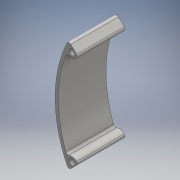
# Autodesk Inventor part: back plate
Saved by Autodesk Inventor 2016 (Build 200138000, 138)
## iProperties
Created: 2015-10-26
Part Number: back plate
Material: Generic
Document SubType Name: Modeling
Designer: Hulbert Office
Density: 1 g/cm^3
Appearance: Default
Author: Hulbert Office
Autodesk Inventor part; units mm, degrees
ref_plane "YZ Plane" through (0, 0, 0) normal (1, 0, 0) x (0, 1, 0)
ref_plane "XZ Plane" through (0, 0, 0) normal (0, 1, 0) x (-1, 0, 0)
ref_plane "XY Plane" through (0, 0, 0) normal (0, 0, 1) x (1, 0, 0)
sketch "Sketch1" plane through (0, 0, 0) normal (0, 1, 0) x (-1, 0, 0)
  line L0 (-57.8698, 32.3928) -> (-57.8698, 32.0292)
  line L1 (-57.8698, 32.0292) -> (-57.8698, 18.4092)
  line L2 (-57.8698, 18.4092) -> (-57.8698, 4.7892)
  line L3 (-57.8698, 4.7892) -> (-57.8698, -8.8308)
  line L4 (-57.8698, -8.8308) -> (-57.8698, -22.4508)
  line L5 (-57.8698, -1.839) -> (-57.8698, -36.0708)
  line L6 (-57.8698, -36.0708) -> (-54.7847, -36.7468)
  line L7 (-54.7847, -36.7468) -> (-50.239, -34.4141)
  line L8 (-50.239, -34.4141) -> (-38.1725, -14.554)
  line L9 (-38.1725, -14.554) -> (-34.8422, -12.8451)
  line L10 (-34.8422, -12.8451) -> (-8.0341, -30.0588)
  line L11 (-8.0341, -30.0588) -> (-8.0341, -78.5822)
  line L12 (-8.0341, -78.5822) -> (-8.0341, -99.6831)
  line L13 (-8.0341, -99.6831) -> (-7.0952, -101.449)
  line L14 (-7.0952, -101.449) -> (-2.0952, -101.449)
  line L15 (-1.1562, -99.6831) -> (-2.0952, -101.449)
  line L16 (-1.1562, -78.5822) -> (-1.1562, -99.6831)
  line L17 (-1.1562, -30.0588) -> (-1.1562, -78.5822)
  line L18 (-1.1562, -30.0588) -> (21.4276, -7.475)
  line L19 (21.4276, -7.475) -> (24.147, -4.7556)
  line L20 (24.147, -4.7556) -> (89.8399, -4.7556)
  line L21 (89.8399, -4.7556) -> (91.6058, -3.8166)
  line L22 (91.6058, 0.1386) -> (91.6058, -3.8166)
  line L23 (89.8399, 1.0776) -> (91.6058, 0.1386)
  line L24 (24.147, 1.0776) -> (89.8399, 1.0776)
  line L25 (21.4276, 3.797) -> (24.147, 1.0776)
  line L26 (-1.1562, 26.3808) -> (21.4276, 3.797)
  line L27 (-1.1562, 26.3808) -> (-1.1562, 74.9042)
  line L28 (-1.1562, 74.9042) -> (-1.1562, 96.0051)
  line L29 (-1.1562, 96.0051) -> (-2.0952, 97.771)
  line L30 (-7.0952, 97.771) -> (-2.0952, 97.771)
  line L31 (-8.0341, 96.0051) -> (-7.0952, 97.771)
  line L32 (-8.0341, 74.9042) -> (-8.0341, 96.0051)
  line L33 (-8.0341, 74.9042) -> (-8.0341, 96.0051)
  line L34 (-8.0341, 26.3808) -> (-8.0341, 74.9042)
  line L35 (-8.0341, 26.3808) -> (-8.0341, 74.9042)
  line L36 (-8.0341, 26.3808) -> (-8.0341, 74.9042)
  line L37 (-8.0341, 26.3808) -> (-8.0341, 74.9042)
  line L38 (-34.8422, 9.1671) -> (-8.0341, 26.3808)
  line L39 (-38.1725, 10.876) -> (-34.8422, 9.1671)
  line L40 (-50.239, 30.7361) -> (-38.1725, 10.876)
  line L41 (-54.7847, 33.0688) -> (-50.239, 30.7361)
  line L42 (-57.8698, 32.3928) -> (-54.7847, 33.0688)
  line L43 (-57.8698, -1.839) -> (-57.8698, -36.0708)
  line L44 (-57.8698, -1.839) -> (-57.8698, -36.0708)
  line L45 (-57.8698, -1.839) -> (-57.8698, -36.0708)
  line L46 (-57.8698, -36.0708) -> (-54.7847, -36.7468)
  line L47 (-54.7847, -36.7468) -> (-50.239, -34.4141)
  line L48 (-50.239, -34.4141) -> (-38.1725, -14.554)
  line L49 (-38.1725, -14.554) -> (-34.8422, -12.8451)
  line L50 (-34.8422, -12.8451) -> (-8.0341, -30.0588)
  line L51 (-8.0341, -30.0588) -> (-8.0341, -78.5822)
  line L52 (-8.0341, -78.5822) -> (-8.0341, -99.6831)
  line L53 (-8.0341, -99.6831) -> (-7.0952, -101.449)
  line L54 (-7.0952, -101.449) -> (-2.0952, -101.449)
  line L55 (-1.1562, -99.6831) -> (-2.0952, -101.449)
  line L56 (-1.1562, -78.5822) -> (-1.1562, -99.6831)
  line L57 (-1.1562, -30.0588) -> (-1.1562, -78.5822)
  line L58 (-1.1562, -30.0588) -> (21.4276, -7.475)
  line L59 (21.4276, -7.475) -> (24.147, -4.7556)
  line L60 (24.147, -4.7556) -> (89.8399, -4.7556)
  line L61 (89.8399, -4.7556) -> (91.6058, -3.8166)
  line L62 (91.6058, 0.1386) -> (91.6058, -3.8166)
  line L63 (89.8399, 1.0776) -> (91.6058, 0.1386)
  line L64 (24.147, 1.0776) -> (89.8399, 1.0776)
  line L65 (21.4276, 3.797) -> (24.147, 1.0776)
  line L66 (-1.1562, 26.3808) -> (21.4276, 3.797)
  line L67 (-1.1562, 26.3808) -> (-1.1562, 74.9042)
  line L68 (-1.1562, 74.9042) -> (-1.1562, 96.0051)
  line L69 (-1.1562, 96.0051) -> (-2.0952, 97.771)
  line L70 (-7.0952, 97.771) -> (-2.0952, 97.771)
  line L71 (-8.0341, 96.0051) -> (-7.0952, 97.771)
  line L72 (-8.0341, 74.9042) -> (-8.0341, 96.0051)
  line L73 (-8.0341, 69.2148) -> (-8.0341, 83.4928)
  line L74 (-8.0341, 54.9368) -> (-8.0341, 69.2148)
  line L75 (-8.0341, 40.6588) -> (-8.0341, 54.9368)
  line L76 (-8.0341, 26.3808) -> (-8.0341, 40.6588)
  line L77 (-34.8422, 9.1671) -> (-8.0341, 26.3808)
  line L78 (-38.1725, 10.876) -> (-34.8422, 9.1671)
  line L79 (-50.239, 30.7361) -> (-38.1725, 10.876)
  line L80 (-54.7847, 33.0688) -> (-50.239, 30.7361)
  line L81 (-57.8698, 32.3928) -> (-54.7847, 33.0688)
  line L82 (-57.8698, 32.3928) -> (-57.8698, 32.0292)
  line L83 (-57.8698, 32.0292) -> (-57.8698, 18.4092)
  line L84 (-57.8698, -1.839) -> (-57.8698, 26.3808)
  line L85 (-57.8698, -1.839) -> (-57.8698, 26.3808)
  line L86 (-8.0341, 26.3808) -> (-8.0341, 40.6588)
  line L87 (-34.8422, 9.1671) -> (-8.0341, 26.3808)
  line L88 (-38.1725, 10.876) -> (-34.8422, 9.1671)
  line L89 (-50.239, 30.7361) -> (-38.1725, 10.876)
  line L90 (-54.7847, 33.0688) -> (-50.239, 30.7361)
  line L91 (-57.8698, 32.3928) -> (-54.7847, 33.0688)
  line L92 (-57.8698, 32.3928) -> (-57.8698, 32.0292)
  line L93 (-57.8698, 32.0292) -> (-57.8698, 18.4092)
  line L94 (-57.8698, -1.839) -> (-57.8698, 26.3808)
  line L95 (-57.8698, -1.839) -> (-57.8698, 26.3808)
  line L96 (-57.8698, -1.839) -> (-57.8698, -36.0708)
  line L97 (-57.8698, -1.839) -> (-57.8698, -36.0708)
  line L98 (-57.8698, -1.839) -> (-57.8698, -36.0708)
  line L99 (-57.8698, -36.0708) -> (-54.7847, -36.7468)
  line L100 (-54.7847, -36.7468) -> (-50.239, -34.4141)
  line L101 (-50.239, -34.4141) -> (-38.1725, -14.554)
  line L102 (-38.1725, -14.554) -> (-34.8422, -12.8451)
  line L103 (-34.8422, -12.8451) -> (-8.0341, -30.0588)
  line L104 (-8.0341, -30.0588) -> (-8.0341, -78.5822)
  line L105 (-8.0341, -78.5822) -> (-8.0341, -99.6831)
  line L106 (-8.0341, -99.6831) -> (-7.0952, -101.449)
  line L107 (-7.0952, -101.449) -> (-2.0952, -101.449)
  line L108 (-1.1562, -99.6831) -> (-2.0952, -101.449)
  line L109 (-1.1562, -78.5822) -> (-1.1562, -99.6831)
  line L110 (-1.1562, -30.0588) -> (-1.1562, -78.5822)
  line L111 (-1.1562, -30.0588) -> (21.4276, -7.475)
  line L112 (21.4276, -7.475) -> (24.147, -4.7556)
  line L113 (24.147, -4.7556) -> (89.8399, -4.7556)
  line L114 (89.8399, -4.7556) -> (91.6058, -3.8166)
  line L115 (91.6058, 0.1386) -> (91.6058, -3.8166)
  line L116 (89.8399, 1.0776) -> (91.6058, 0.1386)
  line L117 (24.147, 1.0776) -> (89.8399, 1.0776)
  line L118 (21.4276, 3.797) -> (24.147, 1.0776)
  line L119 (-1.1562, 26.3808) -> (21.4276, 3.797)
  line L120 (-1.1562, 26.3808) -> (-1.1562, 74.9042)
  line L121 (-1.1562, 74.9042) -> (-1.1562, 96.0051)
  line L122 (-1.1562, 96.0051) -> (-2.0952, 97.771)
  line L123 (-7.0952, 97.771) -> (-2.0952, 97.771)
  line L124 (-8.0341, 96.0051) -> (-7.0952, 97.771)
  line L125 (-8.0341, 74.9042) -> (-8.0341, 96.0051)
  line L126 (-8.0341, 69.2148) -> (-8.0341, 83.4928)
  line L127 (-8.0341, 54.9368) -> (-8.0341, 69.2148)
  line L128 (-8.0341, 26.3808) -> (-8.0341, 74.9042)
  line L129 (-57.8698, -1.839) -> (-57.8698, 26.3808)
  line L130 (-57.8698, -1.839) -> (-57.8698, 26.3808)
  line L131 (-57.8698, -1.839) -> (-57.8698, 26.3808)
  line L132 (-57.8698, -1.839) -> (-57.8698, -36.0708)
  line L133 (-57.8698, -1.839) -> (-57.8698, -36.0708)
  line L134 (-57.8698, -1.839) -> (-57.8698, -36.0708)
  line L135 (-57.8698, -36.0708) -> (-54.7847, -36.7468)
  line L136 (-54.7847, -36.7468) -> (-50.239, -34.4141)
  line L137 (-50.239, -34.4141) -> (-38.1725, -14.554)
  line L138 (-38.1725, -14.554) -> (-34.8422, -12.8451)
  line L139 (-34.8422, -12.8451) -> (-8.0341, -30.0588)
  line L140 (-8.0341, -30.0588) -> (-8.0341, -78.5822)
  line L141 (-8.0341, -78.5822) -> (-8.0341, -99.6831)
  line L142 (-8.0341, -99.6831) -> (-7.0952, -101.449)
  line L143 (-7.0952, -101.449) -> (-2.0952, -101.449)
  line L144 (-1.1562, -99.6831) -> (-2.0952, -101.449)
  line L145 (-1.1562, -78.5822) -> (-1.1562, -99.6831)
  line L146 (-1.1562, -30.0588) -> (-1.1562, -78.5822)
  line L147 (-1.1562, -30.0588) -> (21.4276, -7.475)
  line L148 (21.4276, -7.475) -> (24.147, -4.7556)
  line L149 (24.147, -4.7556) -> (89.8399, -4.7556)
  line L150 (89.8399, -4.7556) -> (91.6058, -3.8166)
  line L151 (91.6058, 0.1386) -> (91.6058, -3.8166)
  line L152 (89.8399, 1.0776) -> (91.6058, 0.1386)
  line L153 (24.147, 1.0776) -> (89.8399, 1.0776)
  line L154 (21.4276, 3.797) -> (24.147, 1.0776)
  line L155 (-1.1562, 26.3808) -> (21.4276, 3.797)
  line L156 (-1.1562, 26.3808) -> (-1.1562, 74.9042)
  line L157 (-1.1562, 74.9042) -> (-1.1562, 96.0051)
  line L158 (-1.1562, 96.0051) -> (-2.0952, 97.771)
  line L159 (-7.0952, 97.771) -> (-2.0952, 97.771)
  line L160 (-8.0341, 96.0051) -> (-7.0952, 97.771)
  line L161 (-8.0341, 74.9042) -> (-8.0341, 96.0051)
  line L162 (-8.0341, 69.2148) -> (-8.0341, 83.4928)
  line L163 (-8.0341, 54.9368) -> (-8.0341, 69.2148)
  line L164 (-8.0341, 40.6588) -> (-8.0341, 54.9368)
  line L165 (-8.0341, 26.3808) -> (-8.0341, 40.6588)
  line L166 (-34.8422, 9.1671) -> (-8.0341, 26.3808)
  line L167 (-38.1725, 10.876) -> (-34.8422, 9.1671)
  line L168 (-50.239, 30.7361) -> (-38.1725, 10.876)
  line L169 (-54.7847, 33.0688) -> (-50.239, 30.7361)
  line L170 (-57.8698, 32.3928) -> (-54.7847, 33.0688)
  line L171 (-57.8698, 32.3928) -> (-57.8698, 32.0292)
  line L172 (-57.8698, 26.3808) -> (-57.8698, 32.0292)
  line L173 (-57.8698, 32.0292) -> (-57.8698, 32.3928)
  line L174 (-57.8698, 32.3928) -> (-54.7847, 33.0688)
  line L175 (-54.7847, 33.0688) -> (-50.239, 30.7361)
  line L176 (-50.239, 30.7361) -> (-38.1725, 10.876)
  line L177 (-38.1725, 10.876) -> (-34.8422, 9.1671)
  line L178 (-34.8422, 9.1671) -> (-8.0341, 26.3808)
  line L179 (-8.0341, 26.3808) -> (-8.0341, 74.9042)
  line L180 (-8.0341, 74.9042) -> (-8.0341, 96.0051)
  line L181 (-8.0341, 96.0051) -> (-7.0952, 97.771)
  line L182 (-7.0952, 97.771) -> (-2.0952, 97.771)
  line L183 (-2.0952, 97.771) -> (-1.1562, 96.0051)
  line L184 (-1.1562, 96.0051) -> (-1.1562, 74.9042)
  line L185 (-1.1562, 74.9042) -> (-1.1562, 26.3808)
  line L186 (-1.1562, 26.3808) -> (21.4276, 3.797)
  line L187 (21.4276, 3.797) -> (24.147, 1.0776)
  line L188 (24.147, 1.0776) -> (89.8399, 1.0776)
  line L189 (89.8399, 1.0776) -> (91.6058, 0.1386)
  line L190 (91.6058, 0.1386) -> (91.6058, -3.8166)
  line L191 (91.6058, -3.8166) -> (89.8399, -4.7556)
  line L192 (89.8399, -4.7556) -> (24.147, -4.7556)
  line L193 (24.147, -4.7556) -> (21.4276, -7.475)
  line L194 (21.4276, -7.475) -> (-1.1562, -30.0588)
  line L195 (-57.8698, 32.0292) -> (-57.8698, 26.3808)
  line L196 (-57.8698, 26.3808) -> (-57.8698, -1.839)
  line L197 (-57.8698, -1.839) -> (-57.8698, -36.0708)
  line L198 (-57.8698, -36.0708) -> (-54.7847, -36.7468)
  line L199 (-54.7847, -36.7468) -> (-50.239, -34.4141)
  line L200 (-50.239, -34.4141) -> (-38.1725, -14.554)
  line L201 (-38.1725, -14.554) -> (-34.8422, -12.8451)
  line L202 (-34.8422, -12.8451) -> (-8.0341, -30.0588)
  line L203 (-8.0341, -30.0588) -> (-8.0341, -78.5822)
  line L204 (-8.0341, -78.5822) -> (-8.0341, -99.6831)
  line L205 (-8.0341, -99.6831) -> (-7.0952, -101.449)
  line L206 (-7.0952, -101.449) -> (-2.0952, -101.449)
  line L207 (-2.0952, -101.449) -> (-1.1562, -99.6831)
  line L208 (-1.1562, -99.6831) -> (-1.1562, -78.5822)
  line L209 (-1.1562, -78.5822) -> (-1.1562, -30.0588)
  line L210 (77.614, -1.839) -> (78.114, -1.839)
  line L211 (78.114, -1.839) -> (78.614, -1.839)
  line L212 (64.1222, -1.839) -> (64.6222, -1.839)
  line L213 (64.6222, -1.839) -> (65.1222, -1.839)
  line L214 (51.6304, -1.839) -> (51.1304, -1.839)
  line L215 (51.1304, -1.839) -> (50.6304, -1.839)
  line L216 (38.1386, -1.839) -> (37.6386, -1.839)
  line L217 (37.6386, -1.839) -> (37.1386, -1.839)
  line L218 (-57.8698, -22.4508) -> (-55.8698, -22.4508)
  line L219 (-55.8698, -22.4508) -> (-55.8698, -22.9508)
  line L220 (-55.8698, -22.4508) -> (-55.8698, -21.9508)
  line L221 (-57.8698, -8.8308) -> (-55.8698, -8.8308)
  line L222 (-55.8698, -8.8308) -> (-55.8698, -9.3308)
  line L223 (-55.8698, -8.8308) -> (-55.8698, -8.3308)
  line L224 (-57.8698, 4.7892) -> (-55.8698, 4.7892)
  line L225 (-55.8698, 4.7892) -> (-55.8698, 4.2892)
  line L226 (-55.8698, 4.7892) -> (-55.8698, 5.2892)
  line L227 (-55.8698, 18.4092) -> (-55.8698, 18.9092)
  line L228 (-55.8698, 18.4092) -> (-55.8698, 17.9092)
  line L229 (-57.8698, 18.4092) -> (-55.8698, 18.4092)
  line L230 (-6.0341, -87.1708) -> (-6.0341, -87.6708)
  line L231 (-6.0341, -44.3368) -> (-6.0341, -43.8368)
  line L232 (-8.0341, -87.1708) -> (-6.0341, -87.1708)
  line L233 (-6.0341, -87.1708) -> (-6.0341, -86.6708)
  line L234 (-6.0341, -72.8928) -> (-6.0341, -73.3928)
  line L235 (-8.0341, -72.8928) -> (-6.0341, -72.8928)
  line L236 (-8.0341, -58.6148) -> (-6.0341, -58.6148)
  line L237 (-6.0341, -44.3368) -> (-6.0341, -44.8368)
  line L238 (-8.0341, -44.3368) -> (-6.0341, -44.3368)
  line L239 (-6.0341, -58.6148) -> (-6.0341, -58.1148)
  line L240 (-6.0341, -58.6148) -> (-6.0341, -59.1148)
  line L241 (-6.0341, -72.8928) -> (-6.0341, -72.3928)
  line L242 (-8.0341, 83.4928) -> (-6.0341, 83.4928)
  line L243 (-6.0341, 83.4928) -> (-6.0341, 82.9928)
  line L244 (-6.0341, 83.4928) -> (-6.0341, 83.9928)
  line L245 (-8.0341, 69.2148) -> (-6.0341, 69.2148)
  line L246 (-6.0341, 69.2148) -> (-6.0341, 68.7148)
  line L247 (-6.0341, 69.2148) -> (-6.0341, 69.7148)
  line L248 (-8.0341, 54.9368) -> (-6.0341, 54.9368)
  line L249 (-6.0341, 54.9368) -> (-6.0341, 54.4368)
  line L250 (-6.0341, 54.9368) -> (-6.0341, 55.4368)
  line L251 (-6.0341, 40.6588) -> (-6.0341, 41.1588)
  line L252 (-6.0341, 40.6588) -> (-6.0341, 40.1588)
  line L253 (-8.0341, 40.6588) -> (-6.0341, 40.6588)
  arc A0 (-93.5154, -61.1235) -> (-93.5154, 57.6128) centre (-175.9423, -1.7554) ccw
  arc A1 (85.0786, -49.2607) -> (85.0786, 45.75) centre (-8.5603, -1.7554) ccw
  arc A2 (-30.2114, -104.4989) -> (38.945, -95.3943) centre (-8.5603, -1.7554) ccw
  line L254 (78.614, -1.839) -> (78.614, -0.439)
  line L255 (78.614, -0.439) -> (83.614, -0.439)
  line L256 (83.614, -0.439) -> (83.614, -3.239)
  line L257 (83.614, -3.239) -> (78.614, -3.239)
  line L258 (78.614, -3.239) -> (78.614, -1.839)
  line L259 (78.114, -1.839) -> (78.114, -1.2219)
  line L260 (77.614, -1.839) -> (77.614, -0.439)
  line L261 (72.614, -3.239) -> (77.614, -3.239)
  line L262 (77.614, -0.439) -> (72.614, -0.439)
  line L263 (72.614, -0.439) -> (72.614, -3.239)
  line L264 (77.614, -3.239) -> (77.614, -1.839)
  line L265 (64.1222, -1.839) -> (64.1222, -0.439)
  line L266 (64.1222, -3.239) -> (64.1222, -1.839)
  line L267 (64.1222, -0.439) -> (59.9222, -0.439)
  line L268 (59.9222, -3.239) -> (64.1222, -3.239)
  line L269 (59.9222, -0.439) -> (59.9222, -3.239)
  line L270 (70.1222, -0.439) -> (70.1222, -3.239)
  line L271 (65.1222, -0.439) -> (70.1222, -0.439)
  line L272 (70.1222, -3.239) -> (65.1222, -3.239)
  line L273 (65.1222, -1.839) -> (65.1222, -0.439)
  line L274 (65.1222, -3.239) -> (65.1222, -1.839)
  line L275 (50.6304, -1.839) -> (50.6304, -0.439)
  line L276 (50.6304, -3.239) -> (50.6304, -1.839)
  line L277 (50.6304, -0.439) -> (46.4304, -0.439)
  line L278 (46.4304, -3.239) -> (50.6304, -3.239)
  line L279 (46.4304, -0.439) -> (46.4304, -3.239)
  line L280 (56.6304, -0.439) -> (56.6304, -3.239)
  line L281 (51.6304, -0.439) -> (56.6304, -0.439)
  line L282 (56.6304, -3.239) -> (51.6304, -3.239)
  line L283 (51.6304, -1.839) -> (51.6304, -0.439)
  line L284 (51.6304, -3.239) -> (51.6304, -1.839)
  line L285 (37.1386, -1.839) -> (37.1386, -0.439)
  line L286 (37.1386, -3.239) -> (37.1386, -1.839)
  line L287 (37.1386, -0.439) -> (32.9386, -0.439)
  line L288 (32.9386, -3.239) -> (37.1386, -3.239)
  line L289 (32.9386, -0.439) -> (32.9386, -3.239)
  line L290 (43.1386, -0.439) -> (43.1386, -3.239)
  line L291 (38.1386, -0.439) -> (43.1386, -0.439)
  line L292 (43.1386, -3.239) -> (38.1386, -3.239)
  line L293 (38.1386, -1.839) -> (38.1386, -0.439)
  line L294 (38.1386, -3.239) -> (38.1386, -1.839)
  line L295 (-6.0341, -59.1148) -> (-3.8341, -59.1148)
  line L296 (-6.0341, -59.1148) -> (-6.0341, -61.4148)
  line L297 (-6.0341, -61.4148) -> (-6.0341, -63.5148)
  line L298 (-3.8341, -67.9148) -> (-3.8341, -59.1148)
  line L299 (-6.0341, -61.4148) -> (-6.0341, -67.9148)
  line L300 (-6.0341, -67.9148) -> (-3.8341, -67.9148)
  line L301 (-6.0341, -43.8368) -> (-5.3341, -43.8368)
  line L302 (-5.3341, -43.8368) -> (-2.7341, -43.8368)
  line L303 (-6.0341, -43.8368) -> (-6.0341, -40.4368)
  line L304 (-6.0341, -40.4368) -> (-2.7341, -40.4368)
  line L305 (-2.7341, -40.4368) -> (-2.7341, -43.8368)
  line L306 (-6.0341, -58.1148) -> (-6.0341, -54.7148)
  line L307 (-6.0341, -58.1148) -> (-5.3341, -58.1148)
  line L308 (-6.0341, -54.7148) -> (-2.7341, -54.7148)
  line L309 (-2.7341, -54.7148) -> (-2.7341, -58.1148)
  line L310 (-5.3341, -58.1148) -> (-2.7341, -58.1148)
  line L311 (-6.0341, -72.3928) -> (-6.0341, -68.9928)
  line L312 (-6.0341, -72.3928) -> (-5.3341, -72.3928)
  line L313 (-6.0341, -68.9928) -> (-2.7341, -68.9928)
  line L314 (-2.7341, -68.9928) -> (-2.7341, -72.3928)
  line L315 (-5.3341, -72.3928) -> (-2.7341, -72.3928)
  line L316 (-6.0341, -86.6708) -> (-6.0341, -83.2708)
  line L317 (-6.0341, -86.6708) -> (-5.3341, -86.6708)
  line L318 (-6.0341, -83.2708) -> (-2.7341, -83.2708)
  line L319 (-2.7341, -83.2708) -> (-2.7341, -86.6708)
  line L320 (-5.3341, -86.6708) -> (-2.7341, -86.6708)
  line L321 (-55.8698, -22.9508) -> (-55.8698, -25.1508)
  line L322 (-55.8698, -25.1508) -> (-53.7698, -25.1508)
  line L323 (-53.7698, -25.1508) -> (-47.1198, -25.1508)
  line L324 (-47.1198, -25.1508) -> (-47.1198, -22.9508)
  line L325 (-47.1198, -22.9508) -> (-55.8698, -22.9508)
  line L326 (-55.8698, -21.9508) -> (-54.8198, -21.9508)
  line L327 (-54.8198, -21.9508) -> (-48.6198, -21.9508)
  line L328 (-55.8698, -21.9508) -> (-55.8698, -20.6508)
  line L329 (-55.8698, -20.6508) -> (-48.6198, -20.6508)
  line L330 (-48.6198, -20.6508) -> (-48.6198, -21.9508)
  line L331 (-6.0341, 40.1588) -> (-6.0341, 36.7588)
  line L332 (-6.0341, 36.7588) -> (-2.9341, 36.7588)
  line L333 (-2.9341, 36.7588) -> (-2.9341, 40.1588)
  line L334 (-2.9341, 40.1588) -> (-6.0341, 40.1588)
  line L335 (-6.0341, -82.1928) -> (-3.8341, -82.1928)
  line L336 (-6.0341, -75.6928) -> (-6.0341, -77.7928)
  line L337 (-6.0341, -75.6928) -> (-6.0341, -82.1928)
  line L338 (-3.8341, -82.1928) -> (-3.8341, -73.3928)
  line L339 (-6.0341, -73.3928) -> (-3.8341, -73.3928)
  line L340 (-6.0341, -73.3928) -> (-6.0341, -75.6928)
  line L341 (-6.0341, -96.4708) -> (-3.8341, -96.4708)
  line L342 (-6.0341, -89.9708) -> (-6.0341, -92.0708)
  line L343 (-6.0341, -89.9708) -> (-6.0341, -96.4708)
  line L344 (-3.8341, -96.4708) -> (-3.8341, -87.6708)
  line L345 (-6.0341, -87.6708) -> (-3.8341, -87.6708)
  line L346 (-6.0341, -87.6708) -> (-6.0341, -89.9708)
  line L347 (-6.0341, -53.6368) -> (-3.8341, -53.6368)
  line L348 (-6.0341, -47.1368) -> (-6.0341, -49.2368)
  line L349 (-6.0341, -47.1368) -> (-6.0341, -53.6368)
  line L350 (-3.8341, -53.6368) -> (-3.8341, -44.8368)
  line L351 (-6.0341, -44.8368) -> (-3.8341, -44.8368)
  line L352 (-6.0341, -44.8368) -> (-6.0341, -47.1368)
  line L353 (-55.8698, -9.3308) -> (-55.8698, -11.5308)
  line L354 (-47.1198, -9.3308) -> (-55.8698, -9.3308)
  line L355 (-47.1198, -11.5308) -> (-47.1198, -9.3308)
  line L356 (-53.7698, -11.5308) -> (-47.1198, -11.5308)
  line L357 (-55.8698, -11.5308) -> (-53.7698, -11.5308)
  line L358 (-54.8198, -8.3308) -> (-48.6198, -8.3308)
  line L359 (-48.6198, -7.0308) -> (-48.6198, -8.3308)
  line L360 (-55.8698, -7.0308) -> (-48.6198, -7.0308)
  line L361 (-55.8698, -8.3308) -> (-55.8698, -7.0308)
  line L362 (-55.8698, -8.3308) -> (-54.8198, -8.3308)
  line L363 (-55.8698, 4.2892) -> (-55.8698, 2.0892)
  line L364 (-47.1198, 4.2892) -> (-55.8698, 4.2892)
  line L365 (-47.1198, 2.0892) -> (-47.1198, 4.2892)
  line L366 (-53.7698, 2.0892) -> (-47.1198, 2.0892)
  line L367 (-55.8698, 2.0892) -> (-53.7698, 2.0892)
  line L368 (-54.8198, 5.2892) -> (-48.6198, 5.2892)
  line L369 (-48.6198, 6.5892) -> (-48.6198, 5.2892)
  line L370 (-55.8698, 6.5892) -> (-48.6198, 6.5892)
  line L371 (-55.8698, 5.2892) -> (-55.8698, 6.5892)
  line L372 (-55.8698, 5.2892) -> (-54.8198, 5.2892)
  line L373 (-55.8698, 17.9092) -> (-55.8698, 15.7092)
  line L374 (-47.1198, 17.9092) -> (-55.8698, 17.9092)
  line L375 (-47.1198, 15.7092) -> (-47.1198, 17.9092)
  line L376 (-53.7698, 15.7092) -> (-47.1198, 15.7092)
  line L377 (-55.8698, 15.7092) -> (-53.7698, 15.7092)
  line L378 (-54.8198, 18.9092) -> (-48.6198, 18.9092)
  line L379 (-48.6198, 20.2092) -> (-48.6198, 18.9092)
  line L380 (-55.8698, 20.2092) -> (-48.6198, 20.2092)
  line L381 (-55.8698, 18.9092) -> (-55.8698, 20.2092)
  line L382 (-55.8698, 18.9092) -> (-54.8198, 18.9092)
  line L383 (-6.0341, 41.1588) -> (-6.0341, 49.8588)
  line L384 (-6.0341, 49.8588) -> (-3.8341, 49.8588)
  line L385 (-3.8341, 49.8588) -> (-3.8341, 41.1588)
  line L386 (-3.8341, 41.1588) -> (-6.0341, 41.1588)
  line L387 (-2.9341, 51.0368) -> (-2.9341, 54.4368)
  line L388 (-6.0341, 54.4368) -> (-6.0341, 51.0368)
  line L389 (-2.9341, 54.4368) -> (-6.0341, 54.4368)
  line L390 (-6.0341, 51.0368) -> (-2.9341, 51.0368)
  line L391 (-3.8341, 55.4368) -> (-6.0341, 55.4368)
  line L392 (-6.0341, 64.1368) -> (-3.8341, 64.1368)
  line L393 (-6.0341, 55.4368) -> (-6.0341, 64.1368)
  line L394 (-3.8341, 64.1368) -> (-3.8341, 55.4368)
  line L395 (-2.9341, 65.3148) -> (-2.9341, 68.7148)
  line L396 (-6.0341, 68.7148) -> (-6.0341, 65.3148)
  line L397 (-2.9341, 68.7148) -> (-6.0341, 68.7148)
  line L398 (-6.0341, 65.3148) -> (-2.9341, 65.3148)
  line L399 (-3.8341, 69.7148) -> (-6.0341, 69.7148)
  line L400 (-6.0341, 78.4148) -> (-3.8341, 78.4148)
  line L401 (-6.0341, 69.7148) -> (-6.0341, 78.4148)
  line L402 (-3.8341, 78.4148) -> (-3.8341, 69.7148)
  line L403 (-2.9341, 79.5928) -> (-2.9341, 82.9928)
  line L404 (-6.0341, 82.9928) -> (-6.0341, 79.5928)
  line L405 (-2.9341, 82.9928) -> (-6.0341, 82.9928)
  line L406 (-6.0341, 79.5928) -> (-2.9341, 79.5928)
  line L407 (-3.8341, 83.9928) -> (-6.0341, 83.9928)
  line L408 (-6.0341, 92.6928) -> (-3.8341, 92.6928)
  line L409 (-6.0341, 83.9928) -> (-6.0341, 92.6928)
  line L410 (-3.8341, 92.6928) -> (-3.8341, 83.9928)
  line L411 (83.614, -1.839) -> (92.364, -1.839)
  line L412 (83.614, -1.839) -> (92.364, -1.839) construction
  arc A3 (81.8808, -49.77) -> (85.0786, -49.2607) centre (83.295, -48.3558) ccw
  line L413 (81.8808, -49.77) -> (71.0762, -38.9655)
  arc A4 (85.0786, -49.2607) -> (85.0786, 45.75) centre (-8.5603, -1.7554) ccw
  line L414 (81.8808, 46.2593) -> (71.0762, 35.4548)
  arc A5 (85.0786, 45.75) -> (81.8808, 46.2593) centre (83.295, 44.8451) ccw
  arc A6 (85.8036, -39.0594) -> (85.8533, 35.4227) centre (-8.5603, -1.7554) ccw
  line L415 (81.4397, -1.7554) -> (81.4397, 38.2446)
  circle A7 centre (81.4397, 38.2446) radius 2.5
  circle A8 centre (81.4397, -41.7554) radius 2.5
  arc A9 (84.4097, -48.9214) -> (84.4097, 45.4107) centre (-8.5603, -1.7554) ccw
  line L416 (84.4097, -48.9214) -> (76.533, -41.0447)
  line L417 (84.4097, 45.4107) -> (76.4785, 37.4794)
  arc A10 (76.4785, 37.4794) -> (85.8533, 35.4227) centre (81.9578, 40.0608) ccw
  arc A11 (85.8533, -39.1007) -> (76.4785, -41.1574) centre (81.9578, -43.7388) ccw
  point P0 (0, 0)
  point P1 (0, 0)
  dimension "d0" = 2.3
  dimension "d1" = 2.1
  dimension "d2" = 6.5
  dimension "d3" = 2.2
  dimension "d4" = 0.7
  dimension "d5" = 2.6
  dimension "d6" = 3.4
  dimension "d7" = 0.7
  dimension "d8" = 2.6
  dimension "d9" = 3.4
  dimension "d10" = 2.6
  dimension "d11" = 3.4
  dimension "d12" = 0.7
  dimension "d13" = 2.6
  dimension "d14" = 3.4
  dimension "d15" = 2.2
  dimension "d16" = 1.3
  dimension "d17" = 3.4
  dimension "d18" = 3.1
  dimension "d19" = 5
  dimension "d20" = 5
  dimension "d21" = 5
  dimension "d22" = 5
  dimension "d23" = 8.8
  dimension "d24" = 2.3
  dimension "d25" = 2.1
  dimension "d26" = 6.5
  dimension "d27" = 2.2
  dimension "d28" = 8.8
  dimension "d29" = 2.3
  dimension "d30" = 2.1
  dimension "d31" = 6.5
  dimension "d32" = 2.2
  dimension "d33" = 8.8
  dimension "d34" = 2.3
  dimension "d35" = 2.1
  dimension "d36" = 6.5
  dimension "d37" = 2.2
  dimension "d38" = 8.8
  dimension "d39" = 8.75
  dimension "d40" = 7.25
  dimension "d41" = 2.2
  dimension "d42" = 1.3
  dimension "d43" = 8.75
  dimension "d44" = 7.25
  dimension "d45" = 2.2
  dimension "d46" = 1.3
  dimension "d47" = 8.75
  dimension "d48" = 7.25
  dimension "d49" = 2.2
  dimension "d50" = 1.3
  dimension "d51" = 8.75
  dimension "d52" = 7.25
  dimension "d53" = 8.7
  dimension "d54" = 2.2
  dimension "d55" = 3.4
  dimension "d56" = 3.1
  dimension "d57" = 8.7
  dimension "d58" = 2.2
  dimension "d59" = 3.4
  dimension "d60" = 3.1
  dimension "d61" = 8.7
  dimension "d62" = 2.2
  dimension "d63" = 3.4
  constraints: 836 end point, 109 point on line, 60 perpendicular, 34 vertical, 30 horizontal, 22 point on circle, 12 centre point, 7 symmetric about line, 5 collinear, 1 coincident, 1 midpoint, 1 parallel, 1 other
  measures "d0" distance of L295.start L296.end
  measures "d1" distance of L296.end L297.end
  measures "d2" distance of L296.end L299.end
  measures "d3" distance of L299.end L298.start
  measures "d4" distance of L231.end L301.end
  measures "d5" distance of L301.end L302.end
  measures "d6" distance of L231.end L303.end
  measures "d7" distance of L306.start L307.end
  measures "d8" distance of L307.end L309.end
  measures "d9" distance of L306.start L306.end
  measures "d10" distance of L312.end L314.end
  measures "d11" distance of L311.start L311.end
  measures "d12" distance of L316.start L317.end
  measures "d13" distance of L317.end L319.end
  measures "d14" distance of L316.start L316.end
  measures "d15" distance of L219.end L321.end
  measures "d16" distance of L220.end L328.end
  measures "d17" distance of L252.end L331.end
  measures "d18" distance of L331.end L332.end
  measures "d19" distance of L256.end L257.end
  measures "d20" distance of L270.end L272.end
  measures "d21" distance of L280.end L282.end
  measures "d22" distance of L290.end L292.end
  measures "d23" distance of L299.end L240.end
  measures "d24" distance of L339.start L336.start
  measures "d25" distance of L336.start L336.end
  measures "d26" distance of L336.start L335.start
  measures "d27" distance of L335.start L335.end
  measures "d28" distance of L335.start point (-6.034, -73.393)
  measures "d29" distance of L345.start L342.start
  measures "d30" distance of L342.start L342.end
  measures "d31" distance of L342.start L341.start
  measures "d32" distance of L341.start L341.end
  measures "d33" distance of L341.start point (-6.034, -87.671)
  measures "d34" distance of L351.start L348.start
  measures "d35" distance of L348.start L348.end
  measures "d36" distance of L348.start L347.start
  measures "d37" distance of L347.start L347.end
  measures "d38" distance of L347.start point (-6.034, -44.837)
  measures "d39" distance of L323.end L321.end
  measures "d40" distance of L329.end L328.end
  measures "d41" distance of L353.start L353.end
  measures "d42" distance of L361.start L360.start
  measures "d43" distance of L355.start L353.end
  measures "d44" distance of L359.start L360.start
  measures "d45" distance of L363.start L363.end
  measures "d46" distance of L371.start L370.start
  measures "d47" distance of L365.start L363.end
  measures "d48" distance of L369.start L370.start
  measures "d49" distance of L373.start L373.end
  measures "d50" distance of L381.start L380.start
  measures "d51" distance of L375.start L373.end
  measures "d52" distance of L379.start L380.start
  measures "d53" distance of L251.end L383.end
  measures "d54" distance of L383.end L384.end
  measures "d55" distance of L388.start L388.end
  measures "d56" distance of L388.end L387.start
  measures "d57" distance of L391.end L392.start
  measures "d58" distance of L392.start L392.end
  measures "d59" distance of L396.start L396.end
  measures "d60" distance of L396.end L395.start
  measures "d61" distance of L399.end L400.start
  measures "d62" distance of L400.start L400.end
  measures "d63" distance of L404.start L404.end
extrude "Extrusion1" add sketch "Sketch1" along normal blind 40 contours A6 A10 L417 A9 L416 A11
fillet "Fillet1" radius 2 6 edges at (-84.4097, 20, -48.9214) (-76.533, 20, -41.0447) (-84.4097, 20, 45.4107) (-85.8533, 20, 35.4227) (-76.4785, 20, 37.4794) (-85.8036, 20, -39.0594)
body "Solid1"
